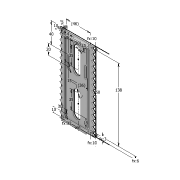
# Autodesk Inventor part: tray
Saved by Autodesk Inventor 2022 (Build 260153000, 153)
## iProperties
Created: 2022-05-19
Part Number: tray
Material: Generic
Document SubType Name: Modeling
Designer: Thomas
Density: 1 g/cm^3
Appearance: Default
Author: Thomas
Autodesk Inventor part; units mm, degrees
ref_plane "YZ Plane" through (0, 0, 0) normal (1, 0, 0) x (0, 1, 0)
ref_plane "XZ Plane" through (0, 0, 0) normal (0, 1, 0) x (-1, 0, 0)
ref_plane "XY Plane" through (0, 0, 0) normal (0, 0, 1) x (1, 0, 0)
sketch "Sketch1" plane through (0, 0, 0) normal (0, 0, 1) x (1, 0, 0)
  line L0 (0, 0) -> (66, 0)
  line L1 (66, 0) -> (66, -150)
  line L2 (66, -150) -> (0, -150)
  line L3 (0, -150) -> (0, 0)
  line L4 (7.6868, 0) -> (92.3291, 0)
  line L5 (9.7325, -150) -> (92.3291, -150)
  line L6 (9.7325, -150) -> (11.7224, -150)
  line L7 (0, 0) -> (5, -5)
  line L8 (0, 0) -> (7.0711, 0) construction
  line L9 (5, -5) -> (0, -10)
  line L10 (0, -10) -> (5, -15)
  line L11 (5, -15) -> (0, -20)
  line L12 (0, -20) -> (5, -25)
  line L13 (5, -25) -> (0, -30)
  line L14 (0, -30) -> (5, -35)
  line L15 (5, -35) -> (0, -40)
  line L16 (0, -40) -> (5, -45)
  line L17 (5, -45) -> (0, -50)
  line L18 (0, -50) -> (5, -55)
  line L19 (5, -55) -> (0, -60)
  line L20 (0, -60) -> (5, -65)
  line L21 (5, -65) -> (0, -70)
  line L22 (0, -70) -> (5, -75)
  line L23 (5, -75) -> (0, -80)
  line L24 (0, -80) -> (5, -85)
  line L25 (5, -85) -> (0, -90)
  line L26 (0, -90) -> (5, -95)
  line L27 (5, -95) -> (0, -100)
  line L28 (0, -100) -> (5, -105)
  line L29 (5, -105) -> (0, -110)
  line L30 (0, -110) -> (5, -115)
  line L31 (5, -115) -> (0, -120)
  line L32 (0, -120) -> (5, -125)
  line L33 (5, -125) -> (0, -130)
  line L34 (0, -130) -> (5, -135)
  line L35 (5, -135) -> (0, -140)
  line L36 (33, 0) -> (33, -140) construction
  line L37 (66, 0) -> (61, -5)
  line L38 (61, -5) -> (66, -10)
  line L39 (66, -10) -> (61, -15)
  line L40 (61, -15) -> (66, -20)
  line L41 (66, -20) -> (61, -25)
  line L42 (61, -25) -> (66, -30)
  line L43 (66, -30) -> (61, -35)
  line L44 (61, -35) -> (66, -40)
  line L45 (66, -40) -> (61, -45)
  line L46 (61, -45) -> (66, -50)
  line L47 (66, -50) -> (61, -55)
  line L48 (61, -55) -> (66, -60)
  line L49 (66, -60) -> (61, -65)
  line L50 (61, -65) -> (66, -70)
  line L51 (66, -70) -> (61, -75)
  line L52 (61, -75) -> (66, -80)
  line L53 (66, -80) -> (61, -85)
  line L54 (61, -85) -> (66, -90)
  line L55 (66, -90) -> (61, -95)
  line L56 (61, -95) -> (66, -100)
  line L57 (66, -100) -> (61, -105)
  line L58 (61, -105) -> (66, -110)
  line L59 (66, -110) -> (61, -115)
  line L60 (61, -115) -> (66, -120)
  line L61 (66, -120) -> (61, -125)
  line L62 (61, -125) -> (66, -130)
  line L63 (66, -130) -> (61, -135)
  line L64 (61, -135) -> (66, -140)
  line L65 (10, -3) -> (56, -3)
  line L66 (56, -3) -> (56, -6)
  line L67 (56, -6) -> (10, -6)
  line L68 (10, -6) -> (10, -3)
  line L69 (10, -144) -> (56, -144)
  line L70 (56, -144) -> (56, -147)
  line L71 (56, -147) -> (10, -147)
  line L72 (10, -147) -> (10, -144)
  line L73 (0, -140) -> (5, -145)
  line L74 (5, -145) -> (0, -150)
  line L75 (61, -5) -> (66, -10)
  line L76 (66, -140) -> (61, -145)
  line L77 (61, -145) -> (66, -150)
  line L78 (11, -10) -> (11, -140) construction
  line L79 (9.4, -10) -> (9.4, -140)
  line L80 (12.6, -140) -> (12.6, -10)
  arc A0 (12.6, -10) -> (9.4, -10) centre (11, -10) ccw
  arc A1 (9.4, -140) -> (12.6, -140) centre (11, -140) ccw
  line L81 (16.5, -40) -> (16.5, -60) construction
  line L82 (15, -40) -> (15, -60)
  line L83 (18, -60) -> (18, -40)
  arc A2 (18, -40) -> (15, -40) centre (16.5, -40) ccw
  arc A3 (15, -60) -> (18, -60) centre (16.5, -60) ccw
  line L84 (49.5, -40) -> (49.5, -60) construction
  line L85 (51, -40) -> (51, -60)
  line L86 (48, -60) -> (48, -40)
  arc A4 (51, -40) -> (48, -40) centre (49.5, -40) ccw
  arc A5 (48, -60) -> (51, -60) centre (49.5, -60) ccw
  line L87 (55, -10) -> (55, -140) construction
  line L88 (56.6, -10) -> (56.6, -140)
  line L89 (53.4, -140) -> (53.4, -10)
  arc A6 (56.6, -10) -> (53.4, -10) centre (55, -10) ccw
  arc A7 (53.4, -140) -> (56.6, -140) centre (55, -140) ccw
  line L90 (33, -129) -> (33, -94) construction
  line L91 (40.5, -129) -> (40.5, -94)
  line L92 (25.5, -94) -> (25.5, -129)
  arc A8 (25.5, -129) -> (40.5, -129) centre (33, -129) ccw
  arc A9 (40.5, -94) -> (25.5, -94) centre (33, -94) ccw
  line L93 (33, -56) -> (33, -21) construction
  line L94 (40.5, -56) -> (40.5, -21)
  line L95 (25.5, -21) -> (25.5, -56)
  arc A10 (25.5, -56) -> (40.5, -56) centre (33, -56) ccw
  arc A11 (40.5, -21) -> (25.5, -21) centre (33, -21) ccw
  point P0 (11, -75)
  point P1 (16.5, -50)
  point P2 (49.5, -50)
  point P3 (55, -75)
  point P4 (33, -111.5)
  point P5 (33, -38.5)
  dimension "d0" = 66
  dimension "d1" = 150
  dimension "d2" = 45
  dimension "d3" = 5
  dimension "d6" = 10
  dimension "d11" = 33
  dimension "d12" = 10
  dimension "d13" = 10
  dimension "d14" = 3
  dimension "d15" = 10
  dimension "d16" = 3
  dimension "d17" = 138
  dimension "d19" = 6
  dimension "d20" = 3.2
  dimension "d21" = 11
  dimension "d22" = 10
  dimension "d23" = 10
  dimension "d24" = 46
  dimension "d25" = 3
  dimension "d26" = 4
  dimension "d27" = 40
  dimension "d28" = 20
  dimension "d29" = 30
  dimension "d30" = 36
  dimension "d36" = 35
  dimension "d37" = 15
  dimension "d38" = 15
  dimension "d39" = 35
  dimension "d40" = 15
  dimension "d41" = 15
  constraints: 204 end point, 59 symmetric about line, 24 point on circle, 16 tangent, 12 centre point, 10 parallel, 9 point on line, 7 horizontal, 5 perpendicular, 4 midpoint, 3 vertical, 1 equal length, 74 other
  measures "d0" distance of L1.end L2.end
  measures "d1" distance of L0.end L1.end
  measures "d2" angle of L7 L8
  measures "d3" horizontal distance of L0.start L7.end
  measures "d6" distance of L0.start L10.start
  measures "d11" distance between parallel lines of L3 L36
  measures "d12" distance between parallel lines of L3 L68
  measures "d13" distance between parallel lines of L1 L66
  measures "d14" distance between parallel lines of L67 L65
  measures "d15" distance between parallel lines of L1 L70
  measures "d16" distance between parallel lines of L69 L71
  measures "d17" distance between parallel lines of L67 L69
  measures "d19" distance between parallel lines of L5 L69
  measures "d20" diameter of A1
  measures "d21" distance between parallel lines of L3 L78
  measures "d22" distance from line of L2 L78.end
  measures "d23" distance from line of L0 L78.start
  measures "d24" distance of L65.start L65.end
  measures "d25" diameter of A3
  measures "d26" distance between parallel lines of L82 L78
  measures "d27" distance from line of L0 L81.start
  measures "d28" distance of L81.start L81.end
  measures "d29" distance between parallel lines of L83 L86
  measures "d30" distance between parallel lines of L85 L82
  measures "d36" distance of L90.start L90.end
  measures "d37" diameter of A9
  measures "d38" distance from line of L69 L90.start
  measures "d39" distance of L93.start L93.end
  measures "d40" diameter of A11
  measures "d41" distance from line of L93.end L67
extrude "Extrusion1" add sketch "Sketch1" along normal blind 2.5 contours L0 L37 L38 L39 L40 L41 L42 L43 L44 L45 L46 L47 L48 L49 L50 L51 L52 L53 L54 L55 L56 L57 L58 L59 L60 L61 L62 L63 L64 L76 L77 L2 L74 L73 L35 L34 L33 L32 L31 L30 L29 L28 L27 L26 L25 L24 L23 L22 L21 L20 L19 L18 L17 L16 L15 L14 L13 L12 L11 L10 L9 L7 | L65 L66 L67 L68 | L69 L70 L71 L72 | A8 L92 A9 L91 | A10 L95 A11 L94
extrude "Extrusion2" add sketch "Sketch1" along normal blind 8 contours L65 L66 L67 L68 | L69 L70 L71 L72
fillet "Fillet1" radius 3 2 edges at (33, -147, 2.5) (33, -3, 2.5)
extrude "Extrusion3" cut sketch "Sketch1" along normal through all contours A8 L92 A9 L91 | A10 L95 A11 L94
equation "\"d11\" = 0.5 * d0"
equation "\"d13\" = d12"
equation "\"d15\" = d12"
equation "\"d16\" = d14"
equation "\"d19\" = -0.5 * d17 + 0.5 * d1"
body "Solid1"
